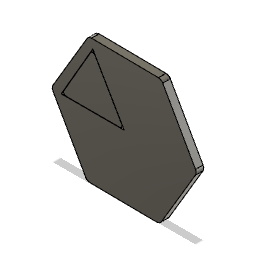
medallion 1 basic with cutout v3 (Autodesk Fusion 360 design; units mm, degrees)
Autodesk Fusion 360 part; units mm, degrees
note: some values were not read from the file. Set by a fixed rule: which sketch regions a step uses.
sketch "Sketch1" plane through (0, 0, 0) normal (0, 0, 1) x (1, 0, 0)
  line L0 (13.5687, 24.844) -> (-12.9876, 25.1527)
  line L1 (-14.7311, 24.1729) -> (-28.2766, 1.3288)
  line L2 (-28.2999, -0.6711) -> (-15.2891, -23.8239)
  line L3 (-13.5687, -24.844) -> (12.9876, -25.1527)
  line L4 (14.7311, -24.1729) -> (28.2766, -1.3288)
  line L5 (28.2999, 0.6711) -> (15.2891, 23.8239)
  arc A0 (-12.9876, 25.1527) -> (-14.7311, 24.1729) centre (-13.0108, 23.1528) ccw
  arc A1 (15.2891, 23.8239) -> (13.5687, 24.844) centre (13.5455, 22.8441) ccw
  arc A2 (28.2766, -1.3288) -> (28.2999, 0.6711) centre (26.5563, -0.3087) ccw
  arc A3 (12.9876, -25.1527) -> (14.7311, -24.1729) centre (13.0108, -23.1528) ccw
  arc A4 (-15.2891, -23.8239) -> (-13.5687, -24.844) centre (-13.5455, -22.8441) ccw
  arc A5 (-28.2766, 1.3288) -> (-28.2999, -0.6711) centre (-26.5563, 0.3087) ccw
  point P0 (-12.5, 7.2169)
  dimension "d1" = 25
  dimension "d7" = 2
  dimension "d8" = 2
  dimension "d9" = 2
  dimension "d10" = 2
  dimension "d11" = 2
  dimension "d12" = 2
  constraint tangent L0 A0
  constraint tangent L1 A0
  constraint tangent L0 A1
  constraint tangent L5 A1
  constraint tangent L4 A2
  constraint tangent L5 A2
  constraint tangent L3 A3
  constraint tangent L4 A3
  constraint tangent L2 A4
  constraint tangent L3 A4
  constraint tangent L1 A5
  constraint tangent L2 A5
  measures "d1" distance of origin L5
  measures "d7" radius of A0
  measures "d8" radius of A1
  measures "d9" radius of A2
  measures "d10" radius of A3
  measures "d11" radius of A4
  measures "d12" radius of A5
extrude "Extrude1" add sketch "Sketch1" along normal blind 3 makes body 1
sketch "Sketch2" plane through (0, 0, 0) normal (0, 0, 1) x (1, 0, 0)
  line L0 (-70.5351, -11.1028) -> (-49.2992, -11.1028)
  line L1 (-48.4332, -9.6028) -> (-59.0511, 8.788)
  line L2 (-60.7832, 8.788) -> (-71.4011, -9.6028)
  arc A0 (-59.0511, 8.788) -> (-60.7832, 8.788) centre (-59.9171, 8.288) ccw
  arc A1 (-49.2992, -11.1028) -> (-48.4332, -9.6028) centre (-49.2992, -10.1028) ccw
  arc A2 (-71.4011, -9.6028) -> (-70.5351, -11.1028) centre (-70.5351, -10.1028) ccw
  point P0 (-47.5671, -11.1028)
  point P1 (-59.9171, 10.288)
  point P2 (-53.3624, 0.343)
  dimension "d16" = 1
  dimension "d17" = 1
  dimension "d21" = 60
  dimension "d22" = 60
  dimension "d24" = 1
  constraint coincident P1 L1
  constraint coincident P1 L2
  constraint tangent L1 A0
  constraint tangent L2 A0
  constraint coincident P0 L0
  constraint coincident P0 L1
  constraint tangent L0 A1
  constraint tangent L1 A1
  constraint tangent L0 A2
  constraint tangent L2 A2
  constraint horizontal L0
  measures "d16" radius of A0
  measures "d17" radius of A1
  measures "d21" angle of L0 L2
  measures "d22" angle of L0 L1
  measures "d24" radius of A2
extrude "Extrude2" add sketch "Sketch2" along normal blind 3 separate body makes body 2
sketch "Sketch4" plane through (0, 0, 3) normal (0, 0, 1) x (1, 0, 0)
  arc A0 (-28.2766, 1.3288) -> (-28.2999, -0.6711) centre (-26.5563, 0.3087) ccw
  line L0 (-28.2999, -0.6711) -> (-15.2891, -23.8239)
  arc A1 (-15.2891, -23.8239) -> (-13.5687, -24.844) centre (-13.5455, -22.8441) ccw
  line L1 (-13.5687, -24.844) -> (12.9876, -25.1527)
  arc A2 (12.9876, -25.1527) -> (14.7311, -24.1729) centre (13.0108, -23.1528) ccw
  line L2 (14.7311, -24.1729) -> (28.2766, -1.3288)
  arc A3 (28.2766, -1.3288) -> (28.2999, 0.6711) centre (26.5563, -0.3087) ccw
  line L3 (28.2999, 0.6711) -> (15.2891, 23.8239)
  arc A4 (15.2891, 23.8239) -> (13.5687, 24.844) centre (13.5455, 22.8441) ccw
  line L4 (13.5687, 24.844) -> (-12.9876, 25.1527)
  arc A5 (-12.9876, 25.1527) -> (-14.7311, 24.1729) centre (-13.0108, 23.1528) ccw
  line L5 (-14.7311, 24.1729) -> (-28.2766, 1.3288)
  line L6 (-12.5, 21.6506) -> (-25, 0)
  line L7 (-25, 0) -> (0, 0)
  line L8 (0, 0) -> (-12.5, 21.6506)
  point P0 (-12.5, 7.2169)
  dimension "d25" = 25
  constraint coincident L7.end L8.start
  constraint horizontal L7
  measures "d25" distance of L6.start L7.end
extrude "Extrude3" cut sketch "Sketch4" against normal up to surface (3 mm away) contours L6 L7 L8 bodies 1
sketch "Sketch5" plane through (0, 0, 3) normal (0, 0, 1) x (1, 0, 0)
  line L0 (-12.5, 21.6506) -> (0, 0)
  line L1 (0, 0) -> (-25, 0)
  line L2 (-25, 0) -> (-12.5, 21.6506)
  arc A0 (-28.2766, 1.3288) -> (-28.2999, -0.6711) centre (-26.5563, 0.3087) ccw
  line L3 (-28.2999, -0.6711) -> (-15.2891, -23.8239)
  arc A1 (-15.2891, -23.8239) -> (-13.5687, -24.844) centre (-13.5455, -22.8441) ccw
  line L4 (-13.5687, -24.844) -> (12.9876, -25.1527)
  arc A2 (12.9876, -25.1527) -> (14.7311, -24.1729) centre (13.0108, -23.1528) ccw
  line L5 (14.7311, -24.1729) -> (28.2766, -1.3288)
  arc A3 (28.2766, -1.3288) -> (28.2999, 0.6711) centre (26.5563, -0.3087) ccw
  line L6 (28.2999, 0.6711) -> (15.2891, 23.8239)
  arc A4 (15.2891, 23.8239) -> (13.5687, 24.844) centre (13.5455, 22.8441) ccw
  line L7 (13.5687, 24.844) -> (-12.9876, 25.1527)
  arc A5 (-12.9876, 25.1527) -> (-14.7311, 24.1729) centre (-13.0108, 23.1528) ccw
  line L8 (-14.7311, 24.1729) -> (-28.2766, 1.3288)
  line L9 (-14.1937, -22.0754) -> (12.7204, -22.0754) construction
  line L10 (12.7204, -22.0754) -> (12.7204, -12.0754) construction
  line L11 (12.7204, -12.0754) -> (-14.1937, -12.0754) construction
  line L12 (-14.1937, -12.0754) -> (-14.1937, -22.0754) construction
  constraint perpendicular L9 L10
  constraint parallel L9 L11
  constraint parallel L10 L12
move_body "Move3" bodies 2 to x (1, 0, 0) y (0, 1, 0) z (0, 0, 1) at (47.42, 11.2, 0)
